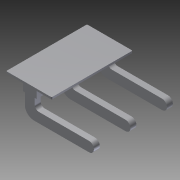
# Autodesk Inventor part: M201230_terminal_angW
Saved by Autodesk Inventor 2011 SP1 (Build 150282100, 282)
## iProperties
Created: 2013-12-24
Part Number: M201230_terminal_angW
Catalog Web Link: www.cadenas.de
Description: Angle Mount Miniature Toggles-terminals-Series M - Miniature Toggles
Vendor: NKKSWITCHES
Document SubType Name: Modeling
Designer: PARTuser1
Manufacturer: NKKSWITCHES
Density: 1 g/cm^3
Category: PARTsolutions
Company: NKKSWITCHES
Title: M201230_terminal_angW
Author: Cadenas PARTsolutions
Comments: Series M - Miniature Toggles
PSOL_IDENT_0: {$CADENAS_DATA\23d-libs\nkkswitches\toggle\m\parts\m_ang_t_terminal.prj},237 {VTYP=3D},{NB=M201230_t
PSOL_IDENT_1: erminal_angW},{LINA=M201230_terminal_angW},{NN=Angle Mount Miniature Toggles-terminals},{DATE=02.06.
PSOL_IDENT_2: 2007 15:25:20},{GEOMDATE=02.06.2007 00:00:00},{VERSION=},{LINEID=10},{LINESUBID=-1},{WBVAR=PLS,CRCTS
PSOL_IDENT_3: ,TRMNLS,CMR}  {NB=M201230_terminal_angW},{LINA=M201230_terminal_angW},{KT=DUMMY},{PN=M201230_termina
PSOL_IDENT_4: l_ang},{SRS=M20},{PLS=1},{CRCTSALG='2','2 - ON/NONE/ON','3','3 - ON/OFF/ON','5','5 - ON/NONE/(ON)','
PSOL_IDENT_5: 8','8 - (ON)/OFF/(ON)','9','9 - ON/OFF/(ON)','4', '4 - ON/ON/ON','6','6 - (ON)/ON/(ON)','7','7 - ON/
PSOL_IDENT_6: ON/(ON)'},{CRCTS=2},{TRMNLSALG='01','01 - Solder Lug','02','02 - Quick Connect','03','03 - .250\" (6
PSOL_IDENT_7: .35mm) Straight PC','05', '05 - .425\" (10.8mm) Wirewrap','06', '06 - .750\" (19.05mm) Wirewrap','07
PSOL_IDENT_8: ', '07 - .964\" (24.5mm) Wirewrap','08', '08 - 1.062\" (27.0mm) Wirewrap'},{TRMNLS=30},{WIDTH=0.512}
PSOL_IDENT_9: ,{HEIGHT=0.37},{LENGTH=0.311},{A=0},{TRMNLNOH=1},{POS=0},{TRMNLOV=3},{D=-0.035},{D2=-0.03500},{M=0.0
PSOL_IDENT_10: 0000},{NUM=0.00000},{TYPE=0.10000},{DSA=0.00000},{CMR=W},{CLR=0.753,0.753,0.753,0.00},{TD=0.10000}
CNS_NN: Angle Mount Miniature Toggles-terminals
CNS_NT: Series M - Miniature Toggles
CNS_NB: M201230_terminal_angW
CNS_NBSYN: $PN.$CMR.
CNS_LINA: M201230_terminal_angW
CNS_PN: M201230_terminal_ang
CNS_SRS: M20
CNS_PLS: 1 - SPST/SPDT
CNS_CRCTSALG: '2','2 - ON/NONE/ON','3','3 - ON/OFF/ON','5','5 - ON/NONE/(ON)','8','8 - (ON)/OFF/(ON)','9','9 - ON/OFF/(ON)','4', '4 - ON/ON/ON','6','6 - (ON)/ON/(ON)','7','7 - ON/ON/(ON)'
CNS_CRCTS: 2 - ON/NONE/ON
CNS_TRMNLSALG: '01','01 - Solder Lug','02','02 - Quick Connect','03','03 - .250" (6.35mm) Straight PC','05', '05 - .425" (10.8mm) Wirewrap','06', '06 - .750" (19.05mm) Wirewrap','07', '07 - .964" (24.5mm) Wirewrap','08', '08 - 1.062" (27.0mm) Wirewrap'
CNS_TRMNLS: 30 - .150" (3.81mm) Right Angle PC (1-3 Pole)
CNS_WIDTH: 0.512
CNS_HEIGHT: 0.370
CNS_LENGTH: 0.311
CNS_A: 0.000
CNS_TRMNLNOH: 1.000
CNS_POS: 0.000
CNS_TRMNLOV: 3.000
CNS_D: -0.035
CNS_D2: -0.03500
CNS_M: 0.00000
CNS_NUM: 0.00000
CNS_TYPE: 0.10000
CNS_DSA: 0.00000
CNS_CMR: W - Silver; Rated 6A @ 125V AC & 3A @ 250V AC
CNS_CLR: 0.753,0.753,0.753,0.00
CNS_TD: 0.10000
SUPPLIER: NKKSWITCHES
ARTICLENO: M201230_terminal_angW
BOMINFO: M201230_terminal_angW
CREATOR: CADENAS GmbH
Autodesk Inventor part; units mm, degrees
sketch "Sketch_2" plane through (0, 0, 0) normal (0, 1, 0) x (-1, 0, 0)
  line L0 (2.9257, -5.0719) -> (2.9257, 5.0719)
  arc A0 (2.9257, 5.0719) -> (2.7957, 5.2019) centre (2.7957, 5.0719) ccw
  line L1 (2.7957, 5.2019) -> (-2.7957, 5.2019)
  arc A1 (-2.7957, 5.2019) -> (-2.9257, 5.0719) centre (-2.7957, 5.0719) ccw
  line L2 (-2.9257, 5.0719) -> (-2.9257, -5.0719)
  arc A2 (-2.9257, -5.0719) -> (-2.7957, -5.2019) centre (-2.7957, -5.0719) ccw
  line L3 (-2.7957, -5.2019) -> (2.7957, -5.2019)
  arc A3 (2.7957, -5.2019) -> (2.9257, -5.0719) centre (2.7957, -5.0719) ccw
  constraints: 8 end point, 8 point on circle, 4 centre point
extrude "Extrusion1" add sketch "Sketch_2" along normal blind 0.254
sketch "Sketch_1" plane through (0, 0, -4.699) normal (0, 0, 1) x (1, 0, 0)
  line L0 (-0.889, 0) -> (-0.889, -1.016)
  line L1 (-0.889, -1.016) -> (-0.635, -1.016)
  line L2 (-0.635, -1.016) -> (-0.635, -2.4384)
  arc A0 (-0.635, -2.4384) -> (0.508, -3.5814) centre (0.508, -2.4384) ccw
  line L3 (0.508, -3.5814) -> (7.6073, -3.5814)
  arc A1 (7.6073, -3.5814) -> (7.6073, -2.3114) centre (7.6073, -2.9464) ccw
  line L4 (7.6073, -2.3114) -> (1.143, -2.3114)
  arc A2 (0.635, -1.8034) -> (1.143, -2.3114) centre (1.143, -1.8034) ccw
  line L5 (0.635, -1.8034) -> (0.635, -1.016)
  line L6 (0.635, -1.016) -> (0.889, -1.016)
  line L7 (0.889, -1.016) -> (0.889, 0)
  line L8 (0.889, 0) -> (-0.889, 0)
  constraints: 18 end point, 6 point on circle, 3 centre point
extrude "Extrusion2" add sketch "Sketch_1" along normal mid plane 0.762
pattern_linear "Rectangular Pattern1" count 3 spacing 4.699 along (0, 0, 1) of "Extrusion2"
ref_plane "to_base_XY" through (0, -0.0254, 0) normal (0, 1, 0) x (1, 0, 0)
ref_plane "to_base_YZ" through (0, -0.0254, 0) normal (1, 0, 0) x (0, 0, -1)
ref_plane "to_base_ZX" through (0, -0.0254, 0) normal (0, 0, -1) x (0, 1, 0)
body "Solid1"
